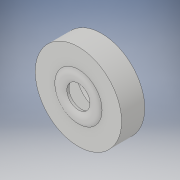
# Autodesk Inventor part: tire 2.2
Saved by Autodesk Inventor 2018.2 (Build 222227000, 227)
## iProperties
Created: 2018-01-27
Part Number: tire 2.2
Material: Generic
Document SubType Name: Modeling
Designer: MIABo
Density: 1 g/cm^3
Appearance: Default
Author: MIABo
Autodesk Inventor part; units mm, degrees
ref_plane "YZ Plane" through (0, 0, 0) normal (1, 0, 0) x (0, 1, 0)
ref_plane "XZ Plane" through (0, 0, 0) normal (0, 1, 0) x (-1, 0, 0)
ref_plane "XY Plane" through (0, 0, 0) normal (0, 0, 1) x (1, 0, 0)
sketch "Sketch1" plane through (0, 0, 0) normal (1, 0, 0) x (0, 1, 0)
  arc A0 (18.2705, 27.94) -> (-10.7536, 27.94) centre (3.7584, 11.6346) ccw
  line L0 (18.2705, 27.94) -> (65.4464, 27.94)
  line L1 (65.4464, 27.94) -> (65.4464, 0)
  line L2 (65.4464, 0) -> (0, 0)
  arc A1 (-10.7536, -27.94) -> (18.2705, -27.94) centre (3.7584, -11.6346) ccw
  line L3 (18.2705, -27.94) -> (65.4464, -27.94)
  line L4 (65.4464, -27.94) -> (65.4464, 0)
  line L5 (-38.6936, 27.94) -> (-38.6936, -27.94)
  line L6 (59.0964, -21.59) -> (15.6101, -21.59)
  line L7 (59.0964, -21.59) -> (59.0964, 21.59)
  line L8 (59.0964, 21.59) -> (15.6101, 21.59)
  arc A2 (15.6101, 21.59) -> (-8.7928, 20.692) centre (3.7584, 11.6346) ccw
  arc A3 (-8.7928, -20.692) -> (15.6101, -21.59) centre (3.7584, -11.6346) ccw
  line L9 (-8.7928, -20.692) -> (-10.7536, -27.94)
  line L10 (-10.7536, 27.94) -> (-8.7928, 20.692)
  dimension "d0" = 27.94
  dimension "d2" = 76.2
  dimension "d3" = 27.94
  dimension "d4" = 6.35
  dimension "d5" = 6.35
  dimension "d6" = 6.35
  dimension "d7" = 6.35
  dimension "d8" = 6.35
  constraints: 22 end point, 8 point on circle, 4 centre point, 4 symmetric about line, 3 horizontal, 2 concentric, 2 perpendicular, 2 vertical, 2 other
  measures "d0" distance of L0.end L1.end
  measures "d2" distance of L10.start L0.end
  measures "d3" distance of L5.end L9.end
  measures "d4" distance between parallel lines of L8 L0
  measures "d5" distance between parallel lines of L3 L6
  measures "d6" radial gap between concentric circles of A1 A3
  measures "d7" radial gap between concentric circles of A2 A0
  measures "d8" distance between parallel lines of L4 L7
revolve "Revolution1" add sketch "Sketch1" angle 360 about axis through (0, -38.6936, 27.94) along (0, 0, -1)
body "Solid1"
